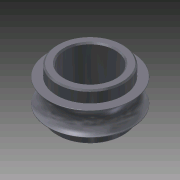
# Autodesk Inventor part: inner ring 1764
Saved by Autodesk Inventor 2011 (Build 150239000, 239)
## iProperties
Created: 2009-01-08
Part Number: inner ring 1764
Document SubType Name: Modeling
Designer: pmulligan
Density: 1 g/cm^3
Author: pmulligan
Autodesk Inventor part; units mm, degrees
ref_plane "YZ Plane" through (0, 0, 0) normal (1, 0, 0) x (0, 1, 0)
ref_plane "XZ Plane" through (0, 0, 0) normal (0, 1, 0) x (-1, 0, 0)
ref_plane "XY Plane" through (0, 0, 0) normal (0, 0, 1) x (1, 0, 0)
sketch "Sketch1" plane through (0, 0, 0) normal (0, 0, 1) x (1, 0, 0)
  line L0 (-25.4863, -2.2875) -> (-25.4863, -4.4623)
  line L1 (-25.4863, -9.0343) -> (-25.4863, -11.209)
  line L2 (-25.4863, -11.209) -> (-23.8988, -11.209)
  line L3 (-23.8988, -11.209) -> (-23.8988, -2.2875)
  line L4 (-23.8988, -2.2875) -> (-25.4863, -2.2875)
  line L5 (-19.1363, -1.7348) -> (-19.1363, -11.209)
  arc A0 (-27.0661, -8.8868) -> (-27.0661, -4.6098) centre (-27.8739, -6.7483) ccw
  line L6 (-27.0392, -9.0343) -> (-25.4863, -9.0343)
  line L7 (-25.4863, -4.4623) -> (-27.0392, -4.4623)
  arc A1 (-27.0392, -4.4623) -> (-27.0661, -4.6098) centre (-27.0392, -4.5385) ccw
  arc A2 (-27.0661, -8.8868) -> (-27.0392, -9.0343) centre (-27.0392, -8.9581) ccw
  dimension "d0" = 2.1747
  dimension "d2" = 2.1747
  dimension "d3" = 1.5875
  dimension "d7" = 4.572
  dimension "d8" = 0.0762
  dimension "d16" = 4.7625
  dimension "d20" = 3.1404
  dimension "d21" = 3.9751
  constraints: 16 end point, 6 point on circle, 6 tangent, 3 centre point, 2 collinear, 2 parallel, 2 perpendicular, 1 equal radius, 1 vertical
  measures "d0" distance of L1.start L1.end
  measures "d2" distance of L0.start L0.end
  measures "d3" distance of L1.end L2.end
  measures "d7" diameter of A0
  measures "d8" radius of A1
  measures "d16" distance between parallel lines of L5 L3
  measures "d20" distance from line of L7.end L3
  measures "d21" distance from line of A0.centre L3
revolve "Revolution1" add sketch "Sketch1" angle 360 about axis through (-19.1363, -1.7348, 0) along (0, -1, 0)
chamfer "Chamfer1" distance 0.254 angle 45 1 edges at (-12.7863, -2.2875, 0)
chamfer "Chamfer2" distance 0.254 angle 45 3 edges at (-14.3738, -2.2875, 0) (-12.7863, -11.209, 0) (-14.3738, -11.209, 0)
body "Solid1"
